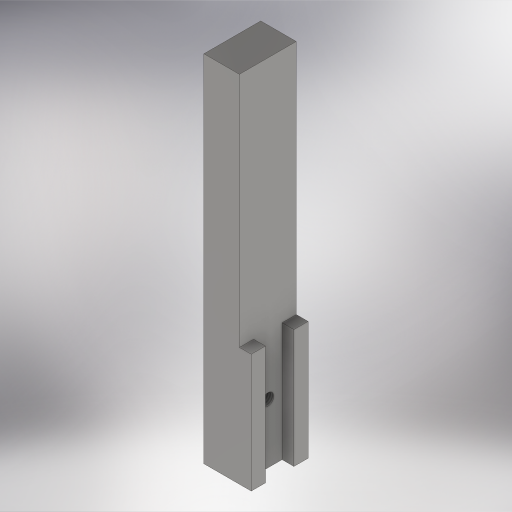
# Autodesk Inventor part: Braço 2
Saved by Autodesk Inventor 2023 (Build 270158000, 158)
## iProperties
Created: 2023-03-17
Part Number: Braço 2
Material: Aço inoxidável
Document SubType Name: Sheet Metal
Designer: Mateus
Density: 8 g/cm^3
Sheet Metal Rule: Padrão_mm
Appearance: Semipolido
Mass: 984 g
Surface Area: 240.8 cm^2
Volume: 123 cm^3
Author: Mateus
Autodesk Inventor part; units mm, degrees
ref_plane "YZ Plane" through (0, 0, 0) normal (1, 0, 0) x (0, 1, 0)
ref_plane "XZ Plane" through (0, 0, 0) normal (0, 1, 0) x (-1, 0, 0)
ref_plane "XY Plane" through (0, 0, 0) normal (0, 0, 1) x (1, 0, 0)
sketch "Esboço1" plane through (0, 0, 0) normal (0, 1, 0) x (-1, 0, 0)
  line L0 (0, 0) -> (15, 0)
  line L1 (15, 0) -> (15, -24)
  line L2 (15, -24) -> (0, -24)
  line L3 (0, -24) -> (0, 0)
  dimension "d0" = 15
  dimension "d1" = 24
  constraints: 8 end point, 2 parallel, 1 horizontal, 1 perpendicular
  measures "d0" distance of L1.end L2.end
  measures "d1" distance of L0.end L1.end
extrude "Extrusão1" add sketch "Esboço1" along normal blind 149.8
sketch "Esboço2" plane through (0, 0, 0) normal (1, 0, 0) x (0, 0, -1)
  line L0 (0, 0) -> (0, 149.8) projected
  line L1 (0, 0) -> (6, 0)
  line L2 (6, 0) -> (6, 50)
  line L3 (6, 50) -> (0, 50)
  line L4 (0, 50) -> (0, 0)
  line L5 (24, 0) -> (0, 0) projected
  line L6 (24, 0) -> (18, 0)
  line L7 (18, 0) -> (18, 50)
  line L8 (18, 50) -> (24, 50)
  line L9 (24, 50) -> (24, 0)
  dimension "d4" = 12
  dimension "d5" = 50
  constraints: 16 end point, 4 parallel, 2 horizontal, 2 perpendicular, 1 collinear, 1 point on line
  measures "d4" distance between parallel lines of L2 L7
  measures "d5" distance of L8.end L5.start
extrude "Extrusão2" add sketch "Esboço2" along normal blind 5
sketch "Esboço3" plane through (-15, 0, -24) normal (-1, 0, 0) x (0, 0, 1)
  line L0 (0, 0) -> (24, 0) projected
  line L1 (24, 0) -> (24, 149.8) projected
  point P0 (12, 25)
  dimension "d8" = 25
  dimension "d9" = 24
  dimension "d10" = 12
  measures "d8" distance from line of L0 point (12, 25)
  measures "d9" distance of L0.start L0.end
  measures "d10" distance from line of L1 point (12, 25)
hole "Furo1" at (-15, 25, -12) direction (1, 0, 0) diameter 4.917 depth 15 tip angle 118 thread size "M6x1" class "6H" standard "ISO Metric profile"
equation "\"d10\" = 0.5 * d9"
equation "\"d16\" = Espessura"
equation "\"Raio_vergadura\" = Espessura"
equation "\"Largura_alívio_de_vergadura\" = Espessura"
equation "\"Profundidade_alívio_de_vergadura\" = 0.5 * Espessura"
equation "\"Tamanho_alívio_de_dobra\" = 4 * Espessura"
equation "\"Remanescente_mínimo\" = 2 * Espessura"
equation "\"Raiodetransição\" = Raio_vergadura"
equation "\"Tamanho_de_raio_de_Jacobi\" = Raio_vergadura"
equation "\"TamanhoFolga\" = Espessura"
equation "\"Espessura\" = 0.5"
